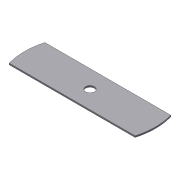
# Autodesk Inventor part: HopperCylinderMount
Saved by Autodesk Inventor 2012 (Build 160160000, 160)
## iProperties
Created: 2013-01-22
Part Number: HopperCylinderMount
Material: Aluminum-6061
Document SubType Name: Modeling
Designer: JesseK
Density: 2.71 g/cm^3
Mass: 179.187 g
Surface Area: 440.061 cm^2
Volume: 66.1206 cm^3
Author: JesseK
Autodesk Inventor part; units mm, degrees
ref_plane "YZ Plane" through (0, 0, 0) normal (1, 0, 0) x (0, 1, 0)
ref_plane "XZ Plane" through (0, 0, 0) normal (0, 1, 0) x (-1, 0, 0)
ref_plane "XY Plane" through (0, 0, 0) normal (0, 0, 1) x (1, 0, 0)
sketch "Sketch2" plane through (0, 0, 0) normal (0, 1, 0) x (-1, 0, 0)
  line L0 (0, 0) -> (268.8083, 0)
  line L1 (268.8083, 76.2) -> (0, 76.2)
  arc A0 (0, 76.2) -> (0, 0) centre (134.4042, 38.1) ccw
  arc A1 (268.8083, 0) -> (268.8083, 76.2) centre (134.4042, 38.1) ccw
  circle A2 centre (134.4042, 38.1) radius 7.9375
  dimension "d0" = 76.2
  dimension "d1" = 139.7
  dimension "d2" = 15.875
  constraints: 4 end point, 4 point on circle, 3 centre point, 2 coincident, 2 parallel, 1 concentric, 1 horizontal
  measures "d0" distance between parallel lines of L0 L1
  measures "d1" radius of A1
  measures "d2" diameter of A2
extrude "Extrusion1" add sketch "Sketch2" along normal blind 3.175
body "Solid1"
